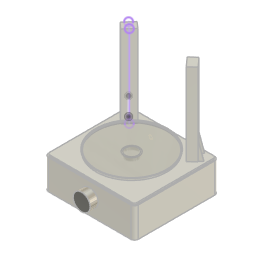
Elegoo Mercury X Cure Station (Autodesk Fusion 360 design; units mm, degrees)
Autodesk Fusion 360 part; units mm, degrees
sketch "Base" plane through (0, 0, 0) normal (0, 0, 1) x (1, 0, 0)
  line L0 (-113, 115) -> (113, 115)
  line L1 (123, 105) -> (123, -105)
  line L2 (113, -115) -> (-113, -115)
  line L3 (-123, -105) -> (-123, 105)
  arc A0 (-113, 115) -> (-123, 105) centre (-113, 105) ccw
  arc A1 (123, 105) -> (113, 115) centre (113, 105) ccw
  arc A2 (113, -115) -> (123, -105) centre (113, -105) ccw
  arc A3 (-123, -105) -> (-113, -115) centre (-113, -105) ccw
  line L4 (-113, 105) -> (113, -105) construction
  dimension "d1" = 10
  dimension "d7" = 246
  dimension "d8" = 230
  constraint horizontal L0
  constraint vertical L1
  constraint horizontal L2
  constraint vertical L3
  constraint tangent L0 A0
  constraint tangent L3 A0
  constraint tangent L0 A1
  constraint tangent L1 A1
  constraint equal A0 A1
  constraint tangent L1 A2
  constraint tangent L2 A2
  constraint equal A0 A2
  constraint tangent L2 A3
  constraint tangent L3 A3
  constraint equal A0 A3
  constraint coincident A0.centre L4.start
  constraint coincident A2.centre L4.end
  constraint midpoint origin L4
  measures "d1" radius of A0
  measures "d7" distance of L1 L3
  measures "d8" distance of L0 L2
extrude "Extrude1" add sketch "Base" along normal blind 81.5 makes body 1
sketch "Base Top" plane through (0, 0, 81.5) normal (0, 0, 1) x (-1, 0, 0)
  arc A0 (113, -115) -> (123, -105) centre (113, -105) ccw
  line L0 (123, -105) -> (123, 105)
  arc A1 (123, 105) -> (113, 115) centre (113, 105) ccw
  line L1 (113, 115) -> (-113, 115)
  arc A2 (-113, 115) -> (-123, 105) centre (-113, 105) ccw
  line L2 (-123, 105) -> (-123, -105)
  arc A3 (-123, -105) -> (-113, -115) centre (-113, -105) ccw
  line L3 (-113, -115) -> (113, -115)
  line L4 (113, 111.5) -> (-113, 111.5)
  arc A4 (-113, 111.5) -> (-119.5, 105) centre (-113, 105) ccw
  line L5 (-119.5, 105) -> (-119.5, -105)
  arc A5 (-119.5, -105) -> (-113, -111.5) centre (-113, -105) ccw
  line L6 (-113, -111.5) -> (113, -111.5)
  arc A6 (113, -111.5) -> (119.5, -105) centre (113, -105) ccw
  line L7 (119.5, -105) -> (119.5, 105)
  arc A7 (119.5, 105) -> (113, 111.5) centre (113, 105) ccw
  dimension "d4" = -3.5
extrude "Extrude2" add sketch "Base Top" along normal blind 4 contours L4 A4 L5 A5 L6 A6 L7 A7 bodies 1
sketch "Wheel" plane through (0, -115, 0) normal (0, -1, 0) x (1, 0, 0)
  line L0 (-113, 0) -> (113, 0)
  line L1 (113, 0) -> (113, 81.5)
  line L2 (113, 81.5) -> (-113, 81.5)
  line L3 (-113, 81.5) -> (-113, 0)
  circle A0 centre (0, 43.15) radius 23.35
  line L4 (0, 66.5) -> (0, 81.5) construction
  dimension "d9" = 46.7
  dimension "d10" = 15
  constraint coincident A0 L4.start
  constraint midpoint L2 L4.end
  constraint vertical L4
  constraint coincident A0.centre L4
  measures "d9" diameter of A0
  measures "d10" distance of L4.start L4.end
extrude "Extrude3" add sketch "Wheel" along normal blind 22 contours A0 bodies 1
sketch "Plate" plane through (0, 0, 0) normal (0, 1, 0) x (1, 0, 0)
  line L0 (20.25, -81.275) -> (20.6, -94.275)
  line L1 (20.6, -94.275) -> (96.966, -94.275)
  line L2 (96.966, -94.275) -> (98.5, -100)
  line L3 (95.3809, -98.405) -> (0, -98.405)
  line L4 (0, -98.405) -> (0, -94.275)
  line L5 (0, -94.275) -> (17.4, -94.275)
  line L6 (17.4, -94.275) -> (17.75, -81.275)
  line L7 (17.75, -81.275) -> (20.25, -81.275)
  line L8 (98.5, -100) -> (95.8083, -100)
  line L9 (95.8083, -100) -> (95.3809, -98.405)
  line L10 (-113, -85.5) -> (113, -85.5)
  dimension "d14" = 98.5
  dimension "d16" = 2.6
  dimension "d17" = 5.725
  dimension "d18" = 4.13
  dimension "d20" = 20.6
  dimension "d23" = 20.25
  dimension "d24" = 2.5
  dimension "d25" = 13
  dimension "d27" = 75
  dimension "d28" = 14.5
  constraint perpendicular L3 L4
  constraint perpendicular L4 L5
  constraint horizontal L8
  constraint parallel L2 L9
  constraint horizontal L7
  constraint coincident L0.end L5
  constraint equal L0 L6
  constraint coincident origin L4
  measures "d14" distance of L4 L2.end
  measures "d16" distance of L2 L9
  measures "d17" distance of L1 L8
  measures "d18" distance of L1 L3
  measures "d20" distance of L0.end L4
  measures "d23" distance of L0.start L4
  measures "d24" distance of L0.start L6.end
  measures "d25" distance of L5.end L7
  measures "d27" angle of L1 L2
  measures "d28" distance of L8 L10
revolve "Revolve1" add sketch "Plate" angle 360 about axis through (0, 0, 98.405) along (0, 0, -1) separate body makes body 2
sketch "Tower" plane through (0, 0, 85.5) normal (0, 0, 1) x (-1, 0, 0)
  arc A0 (119.5, 105) -> (113, 111.5) centre (113, 105) ccw
  line L0 (113, 111.5) -> (-113, 111.5)
  arc A1 (-113, 111.5) -> (-119.5, 105) centre (-113, 105) ccw
  line L1 (-119.5, 105) -> (-119.5, -105)
  arc A2 (-119.5, -105) -> (-113, -111.5) centre (-113, -105) ccw
  line L2 (-113, -111.5) -> (113, -111.5)
  arc A3 (113, -111.5) -> (119.5, -105) centre (113, -105) ccw
  line L3 (119.5, -105) -> (119.5, 105)
  line L4 (89.9753, -59.7376) -> (106.8, -75.4248)
  line L5 (106.8, -75.4248) -> (84.8525, -99.8)
  line L6 (84.8525, -99.8) -> (67.4925, -84.7073)
  line L7 (67.4925, -84.7073) -> (89.9753, -59.7376)
  dimension "d30" = 32.8
  dimension "d31" = 33.6
  dimension "d32" = 23
  dimension "d33" = 12.7
  dimension "d34" = 11.7
  dimension "d36" = 42
  constraint parallel L5 L7
  constraint equal L4 L6
  measures "d30" distance of L4.end L5.end
  measures "d31" distance of L4.start L6.end
  measures "d32" distance of L5 L7
  measures "d33" distance of L3 L4.end
  measures "d34" distance of L2 L5.end
  measures "d36" angle of L3 L5
extrude "Extrude4" add sketch "Tower" along normal blind 225 contours L4 L5 L6 L7 bodies 1
ref_plane "WorkPlane1" through (-87.1728, 79.8208, 198) normal (-0.669131, -0.743145, 0) x (0.743145, -0.669131, 0)
sketch "Tower Support" plane through (0.6614, 0.7346, 0) normal (-0.669131, -0.743145, 0) x (0.743145, -0.669131, 0)
  line L0 (-129.8369, 134.9) -> (-140.8369, 85.5)
  line L1 (-140.8369, 85.5) -> (-129.8369, 85.5)
  line L2 (-129.8369, 85.5) -> (-129.8369, 134.9)
  line L3 (-129.8369, 85.5) -> (-129.8369, 310.5)
  line L4 (-106.8369, 85.5) -> (-106.8369, 310.5)
  dimension "d39" = 34
  dimension "d40" = 49.4
  constraint horizontal L1
  constraint perpendicular L1 L2
  constraint coincident L0.start L3
  constraint coincident L1.end L2.start
  measures "d39" distance of L0.end L4
  measures "d40" distance of L0.start L1.end
extrude "Extrude5" add sketch "Tower Support" along normal mid plane 29 bodies 1
extrude "Extrude6" cut sketch "Tower Support" along normal mid plane 25.5 bodies 1
mirror "Mirror1" about plane through (0, 0, 0) normal (1, 0, 0) of bodies 1 merged
sketch "Power Port" plane through (0, 115, 0) normal (0, 1, 0) x (-1, 0, 0)
  line L0 (-113, 0) -> (113, 0)
  line L1 (113, 0) -> (113, 81.5)
  line L2 (113, 81.5) -> (-113, 81.5)
  line L3 (-113, 81.5) -> (-113, 0)
  circle A0 centre (62.75, 39.95) radius 6.25
  line L4 (62.75, 46.2) -> (62.75, 81.5) construction
  line L5 (69, 39.95) -> (123, 39.95) construction
  line L6 (123, 0) -> (123, 81.5) construction
  circle A1 centre (62.75, 39.95) radius 2.8
  dimension "d47" = 12.5
  dimension "d48" = 35.3
  dimension "d49" = 54
  dimension "d50" = 5.6
  constraint coincident A0 L4.start
  constraint coincident L2 L4.end
  constraint perpendicular L2 L4
  constraint coincident A0.centre L4
  constraint coincident A0 L5.start
  constraint horizontal L5
  constraint coincident L5.end L6
  constraint coincident A0.centre L5
  constraint concentric A0 A1
  measures "d47" diameter of A0
  measures "d48" distance of L4.start L4.end
  measures "d49" distance of L5.start L5.end
  measures "d50" diameter of A1
extrude "Extrude7" add sketch "Power Port" along normal blind 2.1 contours A0 bodies 1
equation "d14 = ( 197 / 2 ) * 1 mm"
equation "d20 = ( 41.2 / 2 ) * 1 mm"
equation "d23 = ( 40.5 / 2 ) * 1 mm"
named bodies: "Main", "Plate"
